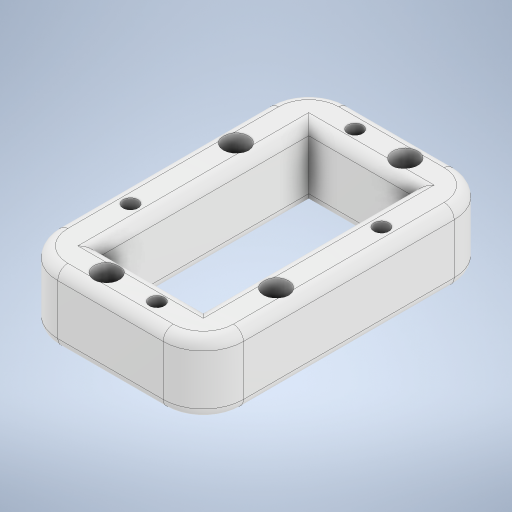
# Autodesk Inventor part: ServoMount
Saved by Autodesk Inventor 2024 (Build 280153000, 153)
## iProperties
Created: 2025-12-19
Part Number: ServoMount
Material: Generic
Document SubType Name: Modeling
Designer: Liam
Density: 1 g/cm^3
Appearance: Default
Mass: 16.4898 g
Surface Area: 85.1058 cm^2
Volume: 16.4898 cm^3
MountWidth: 21.000 mm
MountLength: 42.000 mm
MountThickness: 8.000 mm
TopToPivot: 20.100 mm
Author: Liam
Autodesk Inventor part; units mm, degrees
ref_plane "YZ Plane" through (0, 0, 0) normal (1, 0, 0) x (0, 1, 0)
ref_plane "XZ Plane" through (0, 0, 0) normal (0, 1, 0) x (-1, 0, 0)
ref_plane "XY Plane" through (0, 0, 0) normal (0, 0, 1) x (1, 0, 0)
sketch "Sketch1" plane through (0, 0, 0) normal (0, 1, 0) x (-1, 0, 0)
  line L0 (0, 0) -> (21, 0)
  line L1 (21, 0) -> (21, -42)
  line L2 (21, -42) -> (0, -42)
  line L3 (0, -42) -> (0, 0)
  circle A0 centre (5.5, 3.75) radius 1.5
  line L4 (21, -21) -> (0, -21) construction
  line L5 (29, -50) -> (29, 8)
  line L6 (29, 8) -> (-8, 8)
  line L7 (-8, 8) -> (-8, -50)
  line L8 (-8, -50) -> (29, -50)
  line L9 (10.5, 8) -> (10.5, 0) construction
  line L10 (10.5, 0) -> (10.5, -42) construction
  line L11 (7.25, -42) -> (13.25, -42)
  circle A1 centre (-4, -10.5) radius 2.5
  circle A2 centre (15.5, 3.75) radius 2.5
  circle A3 centre (5.5, -45.75) radius 2.5
  circle A4 centre (15.5, -45.75) radius 1.5
  circle A5 centre (-4, -31.5) radius 1.5
  circle A6 centre (25, -31.5) radius 2.5
  circle A7 centre (25, -10.5) radius 1.5
  circle A8 centre (10.5, -29.9) radius 1
  dimension "d0" = 42
  dimension "d1" = 21
  dimension "d7" = 3
  dimension "d12" = 8
  dimension "d13" = 58
  dimension "d14" = 37
  dimension "d15" = 3.75
  dimension "d16" = 5
  dimension "d35" = 5
  dimension "d36" = 4
  dimension "d37" = 10.5
  dimension "d49" = 5
  dimension "d50" = 3.75
  dimension "d51" = 5
  dimension "d52" = 3.75
  dimension "d53" = 3.75
  dimension "d54" = 5
  dimension "d55" = 5
  dimension "d56" = 5
  dimension "d57" = 3
  dimension "d58" = 10.5
  dimension "d59" = 4
  dimension "d60" = 3
  dimension "d61" = 10.5
  dimension "d62" = 10.5
  dimension "d63" = 4
  dimension "d64" = 4
  dimension "d65" = 3
  dimension "d66" = 5
  dimension "d68" = 2
  dimension "d69" = 20.1
  constraints: 24 end point, 9 centre point, 5 midpoint, 4 parallel, 2 horizontal, 2 perpendicular, 2 point on line, 3 other
  measures "d0" distance of L2.end L0.start
  measures "d1" distance of L0.start L0.end
  measures "d7" diameter of A0
  measures "d12" distance between parallel lines of L1 L5
  measures "d13" distance of L6.end L7.end
  measures "d14" distance of L7.end L5.start
  measures "d15" distance from line of L0 A0.centre
  measures "d16" distance from line of L9 A0.centre
  measures "d35" diameter of A1
  measures "d36" distance from line of L3 A1.centre
  measures "d37" distance from line of L4 A1.centre
  measures "d49" distance from line of L9 A2.centre
  measures "d50" distance from line of L0 A2.centre
  measures "d51" diameter of A2
  measures "d52" distance from line of L2 A3.centre
  measures "d53" distance from line of L2 A4.centre
  measures "d54" distance from line of L10 A4.centre
  measures "d55" distance from line of A3.centre L10
  measures "d56" diameter of A3
  measures "d57" diameter of A4
  measures "d58" distance from line of A5.centre L4
  measures "d59" distance from line of A5.centre L3
  measures "d60" diameter of A5
  measures "d61" distance from line of A7.centre L4
  measures "d62" distance from line of A6.centre L4
  measures "d63" distance from line of L1 A6.centre
  measures "d64" distance from line of L1 A7.centre
  measures "d65" diameter of A7
  measures "d66" diameter of A6
  measures "d68" diameter of A8
  measures "d69" distance from line of L8 A8.centre
extrude "Extrusion1" add sketch "Sketch1" along normal blind 14 contours L8 L7 L6 L5
fillet "Fillet2" radius 8 4 edges at (8, 7, -50) (-29, 7, -50) (-29, 7, 8) (8, 7, 8)
fillet "Fillet3" radius 2 24 edges at (-21, 14, -21) (-10.5, 14, 0) (0, 14, -21) (-10.5, 14, -42) (-10.5, 14, -50) (5.6569, 14, -47.6569) (8, 14, -21) (5.6569, 14, 5.6569) (-10.5, 14, 8) (-26.6569, 14, 5.6569) (-29, 14, -21) (-26.6569, 14, -47.6569) (8, 0, -21) (5.6569, 0, -47.6569) (-10.5, 0, -50) (-26.6569, 0, -47.6569) (-29, 0, -21) (-26.6569, 0, 5.6569) (-10.5, 0, 8) (5.6569, 0, 5.6569) (-21, 0, -21) (-10.5, 0, 0) (0, 0, -21) (-10.5, 0, -42)
equation "\"d0\" = MountLength"
equation "\"d1\" = MountWidth"
equation "\"d12\" = MountThickness"
equation "\"d37\" = 0.25 * MountLength"
equation "\"d58\" = 0.25 * MountLength"
equation "\"d61\" = 0.25 * MountLength"
equation "\"d62\" = 0.25 * MountLength"
equation "\"d25\" = INNER_HEIGHT"
equation "\"MountWidth\" = 21"
equation "\"MountLength\" = 42"
equation "\"MountThickness\" = 8"
equation "\"MountHoleX\" = 5"
equation "\"MountHoleY\" = 3.75"
equation "\"TopToPivot\" = 20.1"
equation "\"INNER_HEIGHT\" = 14"
body "Solid1"
